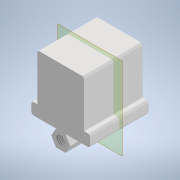
# Autodesk Inventor part: mass
Saved by Autodesk Inventor 2020 (Build 240168000, 168)
## iProperties
Created: 2022-12-14
Part Number: mass
Material: Generic
Document SubType Name: Modeling
Designer: Manish
Density: 1 g/cm^3
Appearance: Default
Author: Manish
Autodesk Inventor part; units mm, degrees
ref_plane "YZ Plane" through (0, 0, 0) normal (1, 0, 0) x (0, 1, 0)
ref_plane "XZ Plane" through (0, 0, 0) normal (0, 1, 0) x (-1, 0, 0)
ref_plane "XY Plane" through (0, 0, 0) normal (0, 0, 1) x (1, 0, 0)
sketch "Sketch1" plane through (0, 0, 0) normal (0, 0, 1) x (1, 0, 0)
  line L0 (2, 0) -> (38, 0)
  line L1 (40, -2) -> (40, -40)
  line L2 (40, -40) -> (0, -40)
  line L3 (0, -40) -> (0, -2)
  line L4 (0, -40) -> (-3, -40)
  line L5 (-5, -42) -> (-5, -48)
  line L6 (-3, -50) -> (43, -50)
  line L7 (45, -48) -> (45, -42)
  line L8 (43, -40) -> (40, -40)
  arc A0 (2, 0) -> (0, -2) centre (2, -2) ccw
  arc A1 (40, -2) -> (38, 0) centre (38, -2) ccw
  arc A2 (-3, -40) -> (-5, -42) centre (-3, -42) ccw
  arc A3 (-5, -48) -> (-3, -50) centre (-3, -48) ccw
  arc A4 (45, -42) -> (43, -40) centre (43, -42) ccw
  arc A5 (43, -50) -> (45, -48) centre (43, -48) ccw
  point P0 (0, 0)
  point P1 (40, 0)
  point P2 (-5, -40)
  point P3 (-5, -50)
  point P4 (45, -50)
  point P5 (45, -40)
  dimension "d0" = 40
  dimension "d1" = 40
  dimension "d2" = 5
  dimension "d3" = 10
  dimension "d4" = 50
  dimension "d5" = 2
  dimension "d6" = 2
  constraints: 18 end point, 13 point on line, 12 point on circle, 12 tangent, 6 centre point, 4 equal radius, 4 perpendicular, 2 horizontal, 2 parallel, 1 collinear
  measures "d0" distance of L1.end L2.end
  measures "d1" distance of point (40, 0) L1.end
  measures "d2" distance of L2.end point (-5, -40)
  measures "d3" distance of point (-5, -40) point (-5, -50)
  measures "d4" distance of point (-5, -50) point (45, -50)
  measures "d5" radius of A0
  measures "d6" radius of A4
extrude "Extrusion1" add sketch "Sketch1" against normal blind 50
sketch "Sketch2" plane through (0, 0, 0) normal (0, 0, 1) x (1, 0, 0)
  line L0 (43, -50) -> (-3, -50) projected
  line L1 (20, -50) -> (20, -57)
  line L2 (-3, -50) -> (43, -50) projected
  circle A0 centre (20, -57) radius 4
  line L3 (24, -50) -> (28.0622, -56.9641)
  line L4 (28.0622, -56.9641) -> (24.0622, -63.9641)
  line L5 (24.0622, -63.9641) -> (16, -64)
  line L6 (16, -64) -> (11.9378, -57.0359)
  line L7 (11.9378, -57.0359) -> (15.9378, -50.0359)
  line L8 (15.9378, -50.0359) -> (24, -50)
  point P0 (0, 0)
  dimension "d9" = 7
  dimension "d10" = 8
  constraints: 14 end point, 2 coincident, 1 centre point, 1 midpoint, 1 perpendicular, 1 point on line, 13 other
  measures "d9" distance of L1.start L1.end
  measures "d10" diameter of A0
extrude "Extrusion2" add sketch "Sketch2" against normal blind 50 contours L3 L4 L5 L6 L7 L8
sketch "Sketch3" plane through (45, -48, 0) normal (1, 0, 0) x (0, 0, -1)
  line L0 (0, 0) -> (0, -2) projected
  line L1 (0, -2) -> (15, -2)
  line L2 (0, -2) -> (50, -2) projected
  line L3 (15, -2) -> (15, -15.9641)
  line L4 (0, -15.9641) -> (50, -15.9641) projected
  line L5 (15, -15.9641) -> (35, -15.9641)
  line L6 (35, -15.9641) -> (35, -2)
  line L7 (15, -2) -> (35, -2)
  point P0 (0, 48)
  dimension "d13" = 15
  dimension "d14" = 20
  constraints: 10 end point, 4 point on line, 1 collinear, 1 perpendicular, 1 vertical
  measures "d13" distance of L0.end L1.end
  measures "d14" distance of L3.end L5.end
extrude "Extrusion3" cut sketch "Sketch3" against normal blind 50
ref_plane "Work Plane1" through (0, 0, -25) normal (0, 0, -1) x (-1, 0, 0)
thread "Thread1" size "M8x1.25" class "6H" standard "ANSI Metric M Profile" full length
thread "Thread2" size "M8x1.25" class "6H" standard "ANSI Metric M Profile" full length
body "Solid1"
